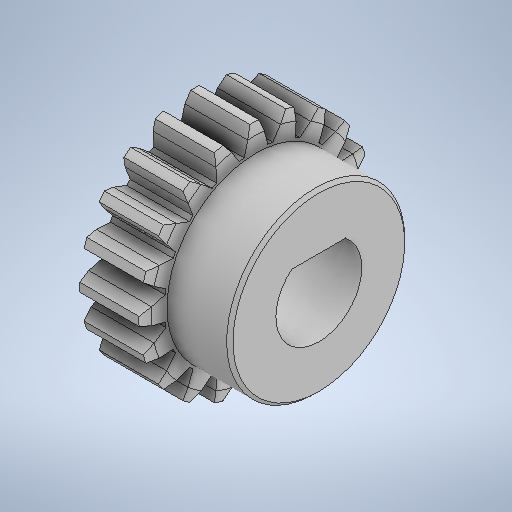
# Autodesk Inventor part: hpc_GG1-20_C
Saved by Autodesk Inventor 2025.2 (Build 292293000, 293)
## iProperties
Category: PARTsolutions
Company: HPC
Created: 2025-05-10
Part Number: hpc_GG1-20_C
Material: Generic
Catalog Web Link: www.cadenas.de
Description: GG 1-Ground spur gear - Heat treated steel - Module 1.0
Vendor: HPC
Document SubType Name: Modeling
Designer: psAdmin
Manufacturer: HPC
Mass: 30 g
Surface Area: 24.0039 cm^2
Volume: 4.25252 cm^3
Density: 1 g/cm^3
Appearance: PSOLRGB-175-175-175
PSOL_IDENT_0: {$CADENAS_DATA/23d-libs/hpc/v4/spur_gear/100/gg1.prj},167 {VTYP=3D},{NB=hpc_GG1-20_C},{LINA=HPC - GG
PSOL_IDENT_1: 1-20},{NN=GG 1},{DATE=17.02.2022 08:08:10},{GEOMDATE=24.09.2019 07:57:00},{VERSION=},{LINEID=2900},{
PSOL_IDENT_2: WBVAR=DET},{WBNUMERIC=}  {NB=hpc_GG1-20_C},{LINA=HPC - GG1-20},{KT=DUMMY},{REF=GG1-20},{DET=C},{Z=20
PSOL_IDENT_3: },{C=20},{D=22},{B=17},{A=6},{J=0.08-0.16},{MAS=0.03},{INFO=INFO},{MODULE=1.000}
NB: hpc_GG1-20_C
NN: GG 1
NT: Ground spur gear - Heat treated steel - Module 1.0
NBSYN: hpc_$REF._$DET.
LINA: HPC - GG1-20
CATALOG: HPC
REF: GG1-20
DET: Full
Z: 20
C: 20
D: 22
B: 17
A: 6
J: 0.08-0.16
MAS: 0.03
INFO: INFO
SUPPLIER: HPC
ARTICLENO: hpc_GG1-20_C
BOMINFO: HPC - GG1-20
CREATOR: CADENAS GmbH
Title: HPC - GG1-20
Author: Cadenas PARTsolutions
Comments: Ground spur gear - Heat treated steel - Module 1.0
Autodesk Inventor part; units mm, degrees
ref_plane "YZ Plane" through (0, 0, 0) normal (1, 0, 0) x (0, 1, 0)
ref_plane "XZ Plane" through (0, 0, 0) normal (0, 1, 0) x (-1, 0, 0)
ref_plane "XY Plane" through (0, 0, 0) normal (0, 0, 1) x (1, 0, 0)
sketch "Esquisse_1" plane through (0, 0, 0) normal (0, 0, 1) x (1, 0, 0)
  line L0 (2, 0) -> (0, 0)
  line L1 (0, 3) -> (12, 3)
  line L2 (12, 3) -> (12, 8.2)
  line L3 (12, 8.2) -> (11.7, 8.5)
  line L4 (11.7, 8.5) -> (6, 8.5)
  line L5 (6, 8.5) -> (6, 10)
  line L6 (6, 10) -> (5.8237, 11)
  line L7 (5.8237, 11) -> (0.1763, 11)
  line L8 (0.1763, 11) -> (0, 10)
  line L9 (0, 10) -> (0, 3)
  point P0 (0, 6.5)
  dimension "d9" = 3
  dimension "d10" = 8
  dimension "d11" = 12
  dimension "d14" = 20
  dimension "d15" = 6
  dimension "d16" = 80
  dimension "d17" = 8.5
  dimension "d20" = 10
  dimension "d21" = 10
  dimension "d22" = 10
  dimension "d24" = 0.3
  dimension "d29" = 135
  constraints: 20 end point, 2 parallel, 1 horizontal, 1 midpoint, 1 point on line, 1 vertical, 1 other
  measures "d9" distance between parallel lines of L0 L1
  measures "d10" distance between parallel lines of L1 L7
  measures "d11" distance between parallel lines of L2 L9
  measures "d14" angle of L6 L8
  measures "d15" distance from line of L5 point (0, 6.5)
  measures "d16" angle of L6 L0
  measures "d17" distance between parallel lines of L4 L0
  measures "d20" distance from line of L5.end L0
  measures "d21" distance from line of L8.end L0
  measures "d22" distance from line of L0.start L2
  measures "d24" horizontal distance of L2.end L3.end
  measures "d29" angle of L2 L3
revolve "Revolution1" add sketch "Esquisse_1" angle 360 about axis through (2, 0, 0) along (1, 0, 0)
sketch "Esquisse_2" plane through (0, 0, 0) normal (1, 0, 0) x (0, 1, 0)
  line L0 (-13, 13) -> (-13, -13)
  line L1 (-13, -13) -> (13, -13)
  line L2 (13, -13) -> (13, 13)
  line L3 (13, 13) -> (-13, 13)
  arc A0 (0.3393, 11.1949) -> (-0.3393, 11.1949) centre (0, 0) ccw
  line L4 (-0.3393, 11.1949) -> (-0.7854, 9.9691)
  line L5 (-0.7854, 9.9691) -> (-1.1318, 8.6765)
  arc A1 (-1.1318, 8.6765) -> (-1.6048, 8.6016) centre (0, 0) ccw
  line L6 (-1.6048, 8.6016) -> (-2.3337, 9.7239)
  line L7 (-2.3337, 9.7239) -> (-3.1367, 10.7518)
  arc A2 (-3.1367, 10.7518) -> (-3.7821, 10.5421) centre (0, 0) ccw
  line L8 (-3.7821, 10.5421) -> (-3.8276, 9.2385)
  line L9 (-3.8276, 9.2385) -> (-3.7575, 7.9021)
  arc A3 (-3.7575, 7.9021) -> (-4.1843, 7.6847) centre (0, 0) ccw
  line L10 (-4.1843, 7.6847) -> (-5.2243, 8.5268)
  line L11 (-5.2243, 8.5268) -> (-6.3057, 9.2562)
  arc A4 (-6.3057, 9.2562) -> (-6.8546, 8.8574) centre (0, 0) ccw
  line L12 (-6.8546, 8.8574) -> (-6.4951, 7.6035)
  line L13 (-6.4951, 7.6035) -> (-6.0155, 6.3542)
  arc A5 (-6.0155, 6.3542) -> (-6.3542, 6.0155) centre (0, 0) ccw
  line L14 (-6.3542, 6.0155) -> (-7.6035, 6.4951)
  line L15 (-7.6035, 6.4951) -> (-8.8574, 6.8546)
  arc A6 (-8.8574, 6.8546) -> (-9.2562, 6.3057) centre (0, 0) ccw
  line L16 (-9.2562, 6.3057) -> (-8.5268, 5.2243)
  line L17 (-8.5268, 5.2243) -> (-7.6847, 4.1843)
  arc A7 (-7.6847, 4.1843) -> (-7.9021, 3.7575) centre (0, 0) ccw
  line L18 (-7.9021, 3.7575) -> (-9.2385, 3.8276)
  line L19 (-9.2385, 3.8276) -> (-10.5421, 3.7821)
  arc A8 (-10.5421, 3.7821) -> (-10.7518, 3.1367) centre (0, 0) ccw
  line L20 (-10.7518, 3.1367) -> (-9.7239, 2.3337)
  line L21 (-9.7239, 2.3337) -> (-8.6016, 1.6048)
  arc A9 (-8.6016, 1.6048) -> (-8.6765, 1.1318) centre (0, 0) ccw
  line L22 (-8.6765, 1.1318) -> (-9.9691, 0.7854)
  line L23 (-9.9691, 0.7854) -> (-11.1949, 0.3393)
  arc A10 (-11.1949, 0.3393) -> (-11.1949, -0.3393) centre (0, 0) ccw
  line L24 (-11.1949, -0.3393) -> (-9.9691, -0.7854)
  line L25 (-9.9691, -0.7854) -> (-8.6765, -1.1318)
  arc A11 (-8.6765, -1.1318) -> (-8.6016, -1.6048) centre (0, 0) ccw
  line L26 (-8.6016, -1.6048) -> (-9.7239, -2.3337)
  line L27 (-9.7239, -2.3337) -> (-10.7518, -3.1367)
  arc A12 (-10.7518, -3.1367) -> (-10.5421, -3.7821) centre (0, 0) ccw
  line L28 (-10.5421, -3.7821) -> (-9.2385, -3.8276)
  line L29 (-9.2385, -3.8276) -> (-7.9021, -3.7575)
  arc A13 (-7.9021, -3.7575) -> (-7.6847, -4.1843) centre (0, 0) ccw
  line L30 (-7.6847, -4.1843) -> (-8.5268, -5.2243)
  line L31 (-8.5268, -5.2243) -> (-9.2562, -6.3057)
  arc A14 (-9.2562, -6.3057) -> (-8.8574, -6.8546) centre (0, 0) ccw
  line L32 (-8.8574, -6.8546) -> (-7.6035, -6.4951)
  line L33 (-7.6035, -6.4951) -> (-6.3542, -6.0155)
  arc A15 (-6.3542, -6.0155) -> (-6.0155, -6.3542) centre (0, 0) ccw
  line L34 (-6.0155, -6.3542) -> (-6.4951, -7.6035)
  line L35 (-6.4951, -7.6035) -> (-6.8546, -8.8574)
  arc A16 (-6.8546, -8.8574) -> (-6.3057, -9.2562) centre (0, 0) ccw
  line L36 (-6.3057, -9.2562) -> (-5.2243, -8.5268)
  line L37 (-5.2243, -8.5268) -> (-4.1843, -7.6847)
  arc A17 (-4.1843, -7.6847) -> (-3.7575, -7.9021) centre (0, 0) ccw
  line L38 (-3.7575, -7.9021) -> (-3.8276, -9.2385)
  line L39 (-3.8276, -9.2385) -> (-3.7821, -10.5421)
  arc A18 (-3.7821, -10.5421) -> (-3.1367, -10.7518) centre (0, 0) ccw
  line L40 (-3.1367, -10.7518) -> (-2.3337, -9.7239)
  line L41 (-2.3337, -9.7239) -> (-1.6048, -8.6016)
  arc A19 (-1.6048, -8.6016) -> (-1.1318, -8.6765) centre (0, 0) ccw
  line L42 (-1.1318, -8.6765) -> (-0.7854, -9.9691)
  line L43 (-0.7854, -9.9691) -> (-0.3393, -11.1949)
  arc A20 (-0.3393, -11.1949) -> (0.3393, -11.1949) centre (0, 0) ccw
  line L44 (0.3393, -11.1949) -> (0.7854, -9.9691)
  line L45 (0.7854, -9.9691) -> (1.1318, -8.6765)
  arc A21 (1.1318, -8.6765) -> (1.6048, -8.6016) centre (0, 0) ccw
  line L46 (1.6048, -8.6016) -> (2.3337, -9.7239)
  line L47 (2.3337, -9.7239) -> (3.1367, -10.7518)
  arc A22 (3.1367, -10.7518) -> (3.7821, -10.5421) centre (0, 0) ccw
  line L48 (3.7821, -10.5421) -> (3.8276, -9.2385)
  line L49 (3.8276, -9.2385) -> (3.7575, -7.9021)
  arc A23 (3.7575, -7.9021) -> (4.1843, -7.6847) centre (0, 0) ccw
  line L50 (4.1843, -7.6847) -> (5.2243, -8.5268)
  line L51 (5.2243, -8.5268) -> (6.3057, -9.2562)
  arc A24 (6.3057, -9.2562) -> (6.8546, -8.8574) centre (0, 0) ccw
  line L52 (6.8546, -8.8574) -> (6.4951, -7.6035)
  line L53 (6.4951, -7.6035) -> (6.0155, -6.3542)
  arc A25 (6.0155, -6.3542) -> (6.3542, -6.0155) centre (0, 0) ccw
  line L54 (6.3542, -6.0155) -> (7.6035, -6.4951)
  line L55 (7.6035, -6.4951) -> (8.8574, -6.8546)
  arc A26 (8.8574, -6.8546) -> (9.2562, -6.3057) centre (0, 0) ccw
  line L56 (9.2562, -6.3057) -> (8.5268, -5.2243)
  line L57 (8.5268, -5.2243) -> (7.6847, -4.1843)
  arc A27 (7.6847, -4.1843) -> (7.9021, -3.7575) centre (0, 0) ccw
  line L58 (7.9021, -3.7575) -> (9.2385, -3.8276)
  line L59 (9.2385, -3.8276) -> (10.5421, -3.7821)
  arc A28 (10.5421, -3.7821) -> (10.7518, -3.1367) centre (0, 0) ccw
  line L60 (10.7518, -3.1367) -> (9.7239, -2.3337)
  line L61 (9.7239, -2.3337) -> (8.6016, -1.6048)
  arc A29 (8.6016, -1.6048) -> (8.6765, -1.1318) centre (0, 0) ccw
  line L62 (8.6765, -1.1318) -> (9.9691, -0.7854)
  line L63 (9.9691, -0.7854) -> (11.1949, -0.3393)
  arc A30 (11.1949, -0.3393) -> (11.1949, 0.3393) centre (0, 0) ccw
  line L64 (11.1949, 0.3393) -> (9.9691, 0.7854)
  line L65 (9.9691, 0.7854) -> (8.6765, 1.1318)
  arc A31 (8.6765, 1.1318) -> (8.6016, 1.6048) centre (0, 0) ccw
  line L66 (8.6016, 1.6048) -> (9.7239, 2.3337)
  line L67 (9.7239, 2.3337) -> (10.7518, 3.1367)
  arc A32 (10.7518, 3.1367) -> (10.5421, 3.7821) centre (0, 0) ccw
  line L68 (10.5421, 3.7821) -> (9.2385, 3.8276)
  line L69 (9.2385, 3.8276) -> (7.9021, 3.7575)
  arc A33 (7.9021, 3.7575) -> (7.6847, 4.1843) centre (0, 0) ccw
  line L70 (7.6847, 4.1843) -> (8.5268, 5.2243)
  line L71 (8.5268, 5.2243) -> (9.2562, 6.3057)
  arc A34 (9.2562, 6.3057) -> (8.8574, 6.8546) centre (0, 0) ccw
  line L72 (8.8574, 6.8546) -> (7.6035, 6.4951)
  line L73 (7.6035, 6.4951) -> (6.3542, 6.0155)
  arc A35 (6.3542, 6.0155) -> (6.0155, 6.3542) centre (0, 0) ccw
  line L74 (6.0155, 6.3542) -> (6.4951, 7.6035)
  line L75 (6.4951, 7.6035) -> (6.8546, 8.8574)
  arc A36 (6.8546, 8.8574) -> (6.3057, 9.2562) centre (0, 0) ccw
  line L76 (6.3057, 9.2562) -> (5.2243, 8.5268)
  line L77 (5.2243, 8.5268) -> (4.1843, 7.6847)
  arc A37 (4.1843, 7.6847) -> (3.7575, 7.9021) centre (0, 0) ccw
  line L78 (3.7575, 7.9021) -> (3.8276, 9.2385)
  line L79 (3.8276, 9.2385) -> (3.7821, 10.5421)
  arc A38 (3.7821, 10.5421) -> (3.1367, 10.7518) centre (0, 0) ccw
  line L80 (3.1367, 10.7518) -> (2.3337, 9.7239)
  line L81 (2.3337, 9.7239) -> (1.6048, 8.6016)
  arc A39 (1.6048, 8.6016) -> (1.1318, 8.6765) centre (0, 0) ccw
  line L82 (1.1318, 8.6765) -> (0.7854, 9.9691)
  line L83 (0.7854, 9.9691) -> (0.3393, 11.1949)
  constraints: 168 end point, 80 point on circle, 40 centre point
extrude "Extrusion1" cut sketch "Esquisse_2" along normal blind 8
sketch "Esquisse6" plane through (12, 0, 0) normal (1, 0, 0) x (0, 0, -1)
  arc A0 (-2.5632, 3.2) -> (2.5632, 3.2) centre (0, 0) ccw
  line L0 (-2.5632, 3.2) -> (2.5632, 3.2)
  dimension "d25" = 8.2
  dimension "d26" = 3.2
  constraints: 2 end point, 2 point on circle, 1 centre point, 1 coincident, 1 horizontal
  measures "d25" diameter of A0
  measures "d26" distance from line of A0.centre L0
extrude "Extrusion5" cut sketch "Esquisse6" against normal through all
body "Solid1"
